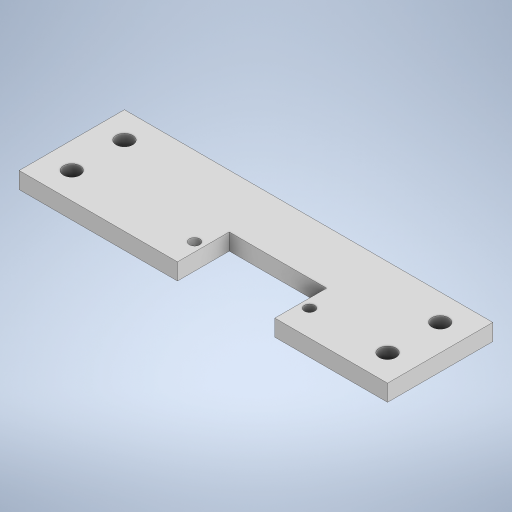
# Autodesk Inventor part: ServoMount
Saved by Autodesk Inventor 2023.1 (Build 271208000, 208)
## iProperties
Created: 2023-05-05
Part Number: ServoMount
Material: Generic
Document SubType Name: Modeling
Designer: bpat387
Density: 1 g/cm^3
Appearance: Default
Author: bpat387
## iProperties of the stored document ServoMount_3DPrint.ipt
Created: 2023-05-05
Part Number: ServoMount_3DPrint
Material: Generic
Document SubType Name: Modeling
Designer: bpat387
Density: 1 g/cm^3
Appearance: Default
Author: bpat387
Autodesk Inventor part; units mm, degrees
ref_plane "YZ Plane" through (0, 0, 0) normal (1, 0, 0) x (0, 1, 0)
ref_plane "XZ Plane" through (0, 0, 0) normal (0, 1, 0) x (-1, 0, 0)
ref_plane "XY Plane" through (0, 0, 0) normal (0, 0, 1) x (1, 0, 0)
sketch "Sketch1" plane through (0, 0, 0) normal (0, 1, 0) x (-1, 0, 0)
  line L0 (0, 0) -> (76.2, 0) construction
  line L1 (76.2, 0) -> (76.2, -25.4) construction
  line L2 (76.2, -25.4) -> (0, -25.4) construction
  line L3 (0, -25.4) -> (0, 0) construction
  line L4 (82.55, -6.35) -> (-6.35, -6.35) construction
  line L5 (-6.35, -6.35) -> (-6.35, -19.05) construction
  line L6 (-6.35, -19.05) -> (82.55, -19.05) construction
  line L7 (82.55, -19.05) -> (82.55, -6.35) construction
  line L8 (-6.35, 0) -> (82.55, 0)
  line L9 (82.55, 0) -> (82.55, -25.4)
  line L10 (82.55, -25.4) -> (-6.35, -25.4)
  line L11 (-6.35, -25.4) -> (-6.35, 0)
  circle A0 centre (76.2, -6.35) radius 2
  circle A1 centre (76.2, -19.05) radius 2
  circle A2 centre (0, -19.05) radius 2
  circle A3 centre (0, -6.35) radius 2
  line L12 (20.8499, 0) -> (44.3499, 0)
  line L13 (44.3499, 0) -> (44.3499, -12.5)
  line L14 (44.3499, -12.5) -> (20.8499, -12.5)
  line L15 (20.8499, -12.5) -> (20.8499, 0)
  line L16 (44.3499, 0) -> (48.5999, 0) construction
  line L17 (48.5999, 0) -> (48.5999, -12.5) construction
  line L18 (48.5999, -12.5) -> (44.3499, -12.5) construction
  line L19 (44.3499, -12.5) -> (44.3499, 0) construction
  line L20 (20.8499, 0) -> (16.5999, 0) construction
  line L21 (16.5999, 0) -> (16.5999, -12.5) construction
  line L22 (16.5999, -12.5) -> (20.8499, -12.5) construction
  line L23 (20.8499, -12.5) -> (20.8499, 0) construction
  line L24 (48.5999, 0) -> (44.3499, -12.5) construction
  line L25 (44.3499, 0) -> (48.5999, -12.5) construction
  line L26 (20.8499, 0) -> (16.5999, -12.5) construction
  line L27 (16.5999, 0) -> (20.8499, -12.5) construction
  circle A4 centre (18.7249, -6.25) radius 1.25
  circle A5 centre (46.4749, -6.25) radius 1.25
  line L28 (44.0999, 0) -> (21.0999, 0) construction
  line L29 (21.0999, 0) -> (21.0999, -12.5) construction
  line L30 (21.0999, -12.5) -> (44.0999, -12.5) construction
  line L31 (44.0999, -12.5) -> (44.0999, 0) construction
  line L32 (44.0999, -6.25) -> (44.3499, -6.25) construction
  line L33 (21.0999, -6.25) -> (20.8499, -6.25) construction
  line L34 (44.0999, 0) -> (38.0999, 0) construction
  line L35 (38.0999, 0) -> (38.0999, -12.5) construction
  line L36 (38.0999, -12.5) -> (44.0999, -12.5) construction
  line L37 (44.0999, -12.5) -> (44.0999, 0) construction
  line L38 (38.0999, -6.25) -> (82.55, -6.25) construction
  line L39 (38.0999, -6.25) -> (-6.35, -6.35) construction
  point P0 (-6.35, -12.7)
  point P1 (82.55, -12.7)
  dimension "d0" = 25.4
  dimension "d1" = 76.2
  dimension "d2" = 12.7
  dimension "d3" = 88.9
  dimension "d4" = 6.35
  dimension "d5" = 6.35
  dimension "d6" = 4
  dimension "d7" = 4
  dimension "d8" = 4
  dimension "d9" = 4
  dimension "d11" = 32
  dimension "d12" = 23.5
  dimension "d13" = 12.5
  dimension "d14" = 2.5
  dimension "d15" = 2.5
  dimension "d16" = 23
  dimension "d17" = 6
  constraints: 80 end point, 18 point on line, 16 parallel, 9 midpoint, 9 perpendicular, 8 horizontal, 6 centre point, 3 equal length
  measures "d0" distance of L0.end L1.end
  measures "d1" distance between parallel lines of L3 L1
  measures "d2" distance of L6.end L4.start
  measures "d3" distance of point (-6.35, -12.7) point (82.55, -12.7)
  measures "d4" distance between parallel lines of L1 L7
  measures "d5" distance between parallel lines of L2 L6
  measures "d6" diameter of A0
  measures "d7" diameter of A1
  measures "d8" diameter of A2
  measures "d9" diameter of A3
  measures "d11" distance between parallel lines of L21 L17
  measures "d12" distance between parallel lines of L23 L13
  measures "d13" distance between parallel lines of L14 L0
  measures "d14" diameter of A4
  measures "d15" diameter of A5
  measures "d16" distance between parallel lines of L29 L31
  measures "d17" distance between parallel lines of L35 L31
extrude "Extrusion1" add sketch "Sketch1" along normal blind 4 contours L8 L15 L14 L13 L9 L10 L11
body "Solid1"
